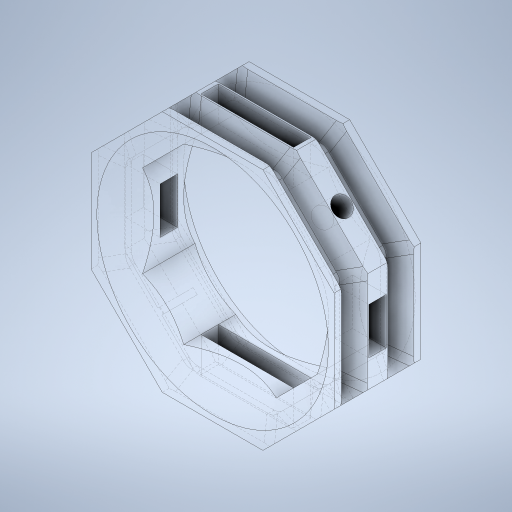
# Autodesk Inventor part: FMR_DXWD80_Helmholtz_Spulenhalter_5mm_OutOfPlane_OCTAGON
Saved by Autodesk Inventor 2023 (Build 270158000, 158)
## iProperties
Created: 2024-01-17
Part Number: FMR_DXWD80_Helmholtz_Spulenhalter_5mm_OutOfPlane_OCTAGON
Material: Generisch
Document SubType Name: Modeling
Designer: Markus Meinert
Density: 1 g/cm^3
Appearance: Vorgabe
Author: Markus Meinert
Autodesk Inventor part; units mm, degrees
ref_plane "YZ Plane" through (0, 0, 0) normal (1, 0, 0) x (0, 1, 0)
ref_plane "XZ Plane" through (0, 0, 0) normal (0, 1, 0) x (-1, 0, 0)
ref_plane "XY Plane" through (0, 0, 0) normal (0, 0, 1) x (1, 0, 0)
sketch "Skizze1" plane through (0, 0, 0) normal (0, 0, 1) x (1, 0, 0)
  line L0 (8.698485, 21) -> (21, 8.698485)
  line L1 (21, 8.698485) -> (21, -8.698485)
  line L2 (21, -8.698485) -> (8.698485, -21)
  line L3 (8.698485, -21) -> (-8.698485, -21)
  line L4 (-8.698485, -21) -> (-21, -8.698485)
  line L5 (-21, -8.698485) -> (-21, 8.698485)
  line L6 (-21, 8.698485) -> (-8.698485, 21)
  line L7 (-8.698485, 21) -> (8.698485, 21)
  point P0 (0, 0)
  point P1 (0, 0)
  dimension "d0" = 21
  constraints: 16 end point, 1 coincident, 17 other
  measures "d0" distance from line of point (0, 0) L7
extrude "Extrusion1" add sketch "Skizze1" along normal mid plane 15
sketch "Skizze2" plane through (0, 0, 7.5) normal (0, 0, 1) x (1, 0, 0)
  circle A0 centre (0, 0) radius 15
  dimension "d3" = 30
  constraints: 1 centre point, 1 coincident
  measures "d3" diameter of A0
extrude "Extrusion2" cut sketch "Skizze2" against normal through all
chamfer "Fase1" distance 5 angle 45 2 edges at (-15, 0, 7.5) (-15, 0, -7.5)
sketch "Skizze3" plane through (0, 0, 0) normal (0, 0, 1) x (1, 0, 0)
  line L0 (6.627417, 16) -> (16, 6.627417)
  line L1 (16, 6.627417) -> (16, -6.627417)
  line L2 (16, -6.627417) -> (6.627417, -16)
  line L3 (6.627417, -16) -> (-6.627417, -16)
  line L4 (-6.627417, -16) -> (-16, -6.627417)
  line L5 (-16, -6.627417) -> (-16, 6.627417)
  line L6 (-16, 6.627417) -> (-6.627417, 16)
  line L7 (-6.627417, 16) -> (6.627417, 16)
  point P0 (0, 0)
  point P1 (0, 0)
  point P2 (0, 16)
  dimension "d43" = 16
  constraints: 16 end point, 1 coincident, 1 midpoint, 17 other
  measures "d43" distance from line of point (0, 0) L7
extrude "Extrusion3" [suppressed]
sketch "Skizze4" plane through (0, 0, 0) normal (0, 1, 0) x (-1, 0, 0)
  line L0 (-21, -7.5) -> (-21, 7.5)
  line L1 (-21, -6.232051) -> (-18, -4.5)
  line L2 (-21, -6.232051) -> (-17.535898, -6.232051) construction
  line L3 (-18, -4.5) -> (-18, -3.5)
  line L4 (-18, -3.5) -> (-21, -1.767949)
  line L5 (-21, 1.767949) -> (-18, 3.5)
  line L6 (-21, 1.767949) -> (-17.535898, 1.767949) construction
  line L7 (-18, 3.5) -> (-18, 4.5)
  line L8 (-18, 4.5) -> (-21, 6.232051)
  line L9 (-18, 4.5) -> (-14.535898, 4.5) construction
  line L10 (-21, -7.5) -> (-21, 7.5)
  point P0 (0, 0)
  point P1 (-21, 0)
  point P2 (-18, -4)
  point P3 (-21, 0)
  point P4 (-18, 4)
  dimension "d11" = 30
  dimension "d12" = 1
  dimension "d13" = 120
  dimension "d14" = 30
  dimension "d15" = 1
  dimension "d16" = 150
  dimension "d17" = 3
  dimension "d18" = 3
  dimension "d19" = 4
  dimension "d20" = 4
  constraints: 18 end point, 4 midpoint, 4 point on line, 3 equal length, 3 horizontal, 1 parallel, 1 vertical
  measures "d11" angle of L2 L1
  measures "d12" distance of L1.end L3.end
  measures "d13" angle of L4 L3
  measures "d14" angle of L6 L5
  measures "d15" distance of L5.end L7.end
  measures "d16" angle of L9 L8
  measures "d17" distance between parallel lines of L0 L3
  measures "d18" distance between parallel lines of L0 L7
  measures "d19" vertical distance of point (-21, 0) point (-18, -4)
  measures "d20" vertical distance of point (-21, 0) point (-18, 4)
sketch3d "3D-Skizze1"
  line L0 (21, -8.698485, 7.5) -> (21, 8.698485, 7.5)
  line L1 (21, 8.698485, 7.5) -> (8.698485, 21, 7.5)
  line L2 (8.698485, 21, 7.5) -> (-8.698485, 21, 7.5)
  line L3 (-8.698485, 21, 7.5) -> (-21, 8.698485, 7.5)
  line L4 (-21, 8.698485, 7.5) -> (-21, -8.698485, 7.5)
  line L5 (-21, -8.698485, 7.5) -> (-8.698485, -21, 7.5)
  line L6 (-8.698485, -21, 7.5) -> (8.698485, -21, 7.5)
  line L7 (8.698485, -21, 7.5) -> (21, -8.698485, 7.5)
sweep "Sweeping1" cut profiles "Skizze4" path "3D-Skizze1"
sketch "Skizze5" plane through (0, 0, 0) normal (0, 1, 0) x (-1, 0, 0)
  line L0 (8, 1.5) -> (-8, 1.5)
  line L1 (-8, 1.5) -> (-8, -1.5)
  line L2 (-8, -1.5) -> (8, -1.5)
  line L3 (8, -1.5) -> (8, 1.5)
  line L4 (8, 1.5) -> (-8, -1.5) construction
  line L5 (-8, 1.5) -> (8, -1.5) construction
  point P0 (0, 0)
  dimension "d23" = 16
  dimension "d24" = 3
  constraints: 12 end point, 2 midpoint, 2 parallel, 1 horizontal, 1 perpendicular
  measures "d23" distance of L2.end L1.end
  measures "d24" distance of L1.end L0.end
extrude "Extrusion4" cut sketch "Skizze5" along normal through all both and the other way through all
sketch "Skizze6" plane through (0, 0, 0) normal (1, 0, 0) x (0, 1, 0)
  line L0 (-4, 1.5) -> (4, 1.5)
  line L1 (4, 1.5) -> (4, -1.5)
  line L2 (4, -1.5) -> (-4, -1.5)
  line L3 (-4, -1.5) -> (-4, 1.5)
  line L4 (-4, 1.5) -> (4, -1.5) construction
  line L5 (4, 1.5) -> (-4, -1.5) construction
  point P0 (0, 0)
  dimension "d27" = 8
  dimension "d28" = 3
  constraints: 12 end point, 2 midpoint, 2 parallel, 1 horizontal, 1 perpendicular
  measures "d27" distance of L1.end L2.end
  measures "d28" distance of L0.end L1.end
extrude "Extrusion5" cut sketch "Skizze6" along normal through all both and the other way through all
sketch "Skizze7" plane through (8.698485, -21, 1.767949) normal (0.7071068, -0.7071068, 0) x (-0.7071068, -0.7071068, 0)
  circle A0 centre (-8.698485, 1.767949) radius 1.6
  dimension "d31" = 3.2
  constraints: 1 centre point, 1 coincident
  measures "d31" diameter of A0
extrude "Extrusion6" cut sketch "Skizze7" against normal blind 5
pattern_circular "Runde Anordnung1" count 2 over 90 about axis through (0, 0, -10) along (0, 0, 1) of "Extrusion6"
fillet "Rundung1" radius 2 16 edges at (-7.4558, 18, -4) (-18, 7.4558, -4) (-18, -7.4558, -4) (-7.4558, -18, -4) (7.4558, -18, -4) (18, -7.4558, -4) (18, 7.4558, -4) (7.4558, 18, -4) (-7.4558, 18, 4) (7.4558, 18, 4) (18, 7.4558, 4) (18, -7.4558, 4) (7.4558, -18, 4) (-7.4558, -18, 4) (-18, -7.4558, 4) (-18, 7.4558, 4)
fillet "Rundung2" radius 5 32 edges at (19.4239, 8.0456, -5.3221) (19.4239, 8.0456, -2.6779) (19.4239, -8.0456, -5.3221) (19.4239, -8.0456, -2.6779) (8.0456, -19.4239, -5.3221) (8.0456, -19.4239, -2.6779) (-8.0456, -19.4239, -5.3221) (-8.0456, -19.4239, -2.6779) (-19.4239, -8.0456, -5.3221) (-19.4239, -8.0456, -2.6779) (-19.4239, 8.0456, -5.3221) (-19.4239, 8.0456, -2.6779) (-8.0456, 19.4239, -5.3221) (-8.0456, 19.4239, -2.6779) (8.0456, 19.4239, -5.3221) (8.0456, 19.4239, -2.6779) (19.4239, 8.0456, 2.6779) (19.4239, 8.0456, 5.3221) (19.4239, -8.0456, 5.3221) (19.4239, -8.0456, 2.6779) (8.0456, -19.4239, 2.6779) (8.0456, -19.4239, 5.3221) (-8.0456, -19.4239, 2.6779) (-8.0456, -19.4239, 5.3221) (-19.4239, -8.0456, 2.6779) (-19.4239, -8.0456, 5.3221) (-19.4239, 8.0456, 2.6779) (-19.4239, 8.0456, 5.3221) (-8.0456, 19.4239, 2.6779) (-8.0456, 19.4239, 5.3221) (8.0456, 19.4239, 2.6779) (8.0456, 19.4239, 5.3221)
sketch "Skizze8" plane through (-21, -8.698485, 1.661275) normal (-0.7071068, -0.7071068, 0) x (-0.7071068, 0.7071068, 0)
  line L0 (-9.198485, -2.338725) -> (-8.198485, -2.338725)
  line L1 (-8.198485, -2.338725) -> (-8.198485, 5.661275)
  line L2 (-8.198485, 5.661275) -> (-9.198485, 5.661275)
  line L3 (-9.198485, 5.661275) -> (-9.198485, -2.338725)
  line L4 (-9.198485, -2.338725) -> (-8.198485, 5.661275) construction
  line L5 (-8.198485, -2.338725) -> (-9.198485, 5.661275) construction
  point P0 (-8.698485, 1.661275)
  dimension "d39" = 1
  dimension "d40" = 8
  constraints: 12 end point, 2 midpoint, 2 parallel, 1 horizontal, 1 perpendicular
  measures "d39" distance of L2.end L1.end
  measures "d40" distance of L1.end L0.end
extrude "Extrusion7" cut sketch "Skizze8" against normal blind 2
sketch "Skizze9" plane through (0, 0, 0) normal (0, 0, 1) x (1, 0, 0)
  line L0 (15.167502, 7.832498) -> (8, 15)
  line L1 (8, 15) -> (-8, 15)
  line L2 (-8, 15) -> (-15.071068, 7.928932)
  line L3 (-15.071068, 7.928932) -> (-15.071068, -7.928932)
  line L4 (-15.071068, -7.928932) -> (-8, -15)
  line L5 (-8, -15) -> (8, -15)
  line L6 (8, -15) -> (15.167502, -7.832498)
  line L7 (15.167502, -7.832498) -> (15.167502, 7.832498)
  circle A0 centre (0, 0) radius 15
  point P0 (0, -15)
  point P1 (0, 15)
  point P2 (-15.071068, 0)
  point P3 (15.167502, 0)
  dimension "d44" = 135
  dimension "d45" = 135
  dimension "d46" = 135
  dimension "d47" = 16
  dimension "d54" = 30
  dimension "d55" = 10
  constraints: 16 end point, 4 midpoint, 4 perpendicular, 2 horizontal alignment, 2 vertical alignment, 1 horizontal, 1 tangent
  measures "d44" angle of L2 L1
  measures "d45" angle of L6 L5
  measures "d46" angle of L1 L0
  measures "d47" distance of L0.end L1.end
  measures "d54" distance between parallel lines of L5 L1
  measures "d55" distance of L1.end L2.end
extrude "Extrusion8" cut sketch "Skizze9" along normal through all both and the other way through all
